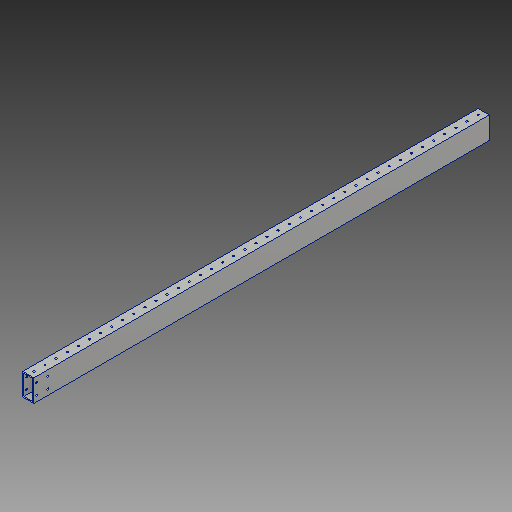
# Autodesk Inventor part: elevator_12''_frame
Saved by Autodesk Inventor 2018 (Build 220112000, 112)
## iProperties
Created: 2018-07-13
Part Number: elevator_12''_frame
Material: Aluminum 6061
Document SubType Name: Modeling
Designer: baoan
Density: 2.7 g/cm^3
Appearance: Aluminum - Flat
Author: baoan
Autodesk Inventor part; units mm, degrees
ref_plane "YZ Plane" through (0, 0, 0) normal (1, 0, 0) x (0, 1, 0)
ref_plane "XZ Plane" through (0, 0, 0) normal (0, 1, 0) x (-1, 0, 0)
ref_plane "XY Plane" through (0, 0, 0) normal (0, 0, 1) x (1, 0, 0)
sketch "Sketch1" plane through (0, 0, 0) normal (0, 0, 1) x (1, 0, 0)
  line L0 (12.7, -25.4) -> (-12.7, -25.4)
  line L1 (-12.7, -25.4) -> (-12.7, 25.4)
  line L2 (-12.7, 25.4) -> (12.7, 25.4)
  line L3 (12.7, 25.4) -> (12.7, -25.4)
  line L4 (12.7, -25.4) -> (-12.7, 25.4) construction
  line L5 (-12.7, -25.4) -> (12.7, 25.4) construction
  line L6 (10.16, -22.86) -> (-10.16, -22.86)
  line L7 (-10.16, -22.86) -> (-10.16, 22.86)
  line L8 (-10.16, 22.86) -> (10.16, 22.86)
  line L9 (10.16, 22.86) -> (10.16, -22.86)
  line L10 (10.16, -22.86) -> (-10.16, 22.86) construction
  line L11 (-10.16, -22.86) -> (10.16, 22.86) construction
  point P0 (0, 0)
  dimension "d0" = 25.4
  dimension "d1" = 50.8
  dimension "d2" = 20.32
  dimension "d3" = 45.72
  constraints: 24 end point, 4 midpoint, 4 parallel, 2 horizontal, 2 perpendicular
  measures "d0" distance of L1.end L2.end
  measures "d1" distance of L0.end L1.end
  measures "d2" distance of L7.end L8.end
  measures "d3" distance of L6.end L7.end
extrude "Extrusion1" add sketch "Sketch1" along normal mid plane 1041.4
sketch "Sketch2" plane through (-12.7, 25.4, 520.7) normal (0, 1, 0) x (1, 0, 0)
  line L0 (0, 0) -> (0, 1041.4) projected
  line L1 (25.4, 0) -> (0, 0) projected
  point P0 (12.7, 520.7)
  point P1 (12.7, 12.7)
  dimension "d6" = 12.7
  dimension "d7" = 12.7
  measures "d6" distance from line of L0 point (12.7, 12.7)
  measures "d7" distance from line of L1 point (12.7, 12.7)
hole "Hole1" at (0, 25.4, 508) direction (0, -1, 0) diameter 4.1402 end through all
pattern_linear "Rectangular Pattern1" count 41 spacing 25.4 along (0, 0, -1) of "Hole1"
sketch "Sketch3" plane through (12.7, -25.4, 520.7) normal (1, 0, 0) x (0, 0, -1)
  line L0 (0, 50.8) -> (1041.4, 50.8) projected
  line L1 (0, 0) -> (0, 50.8) projected
  point P0 (520.7, 25.4)
  point P1 (6.35, 38.1)
  point P2 (6.35, 12.7)
  point P3 (31.75, 38.1)
  point P4 (31.75, 12.7)
  dimension "d18" = 12.7
  dimension "d19" = 25.4
  dimension "d20" = 25.4
  dimension "d22" = 25.4
  dimension "d23" = 6.35
  constraints: 2 vertical alignment, 1 horizontal alignment
  measures "d18" distance from line of L0 point (6.35, 38.1)
  measures "d19" distance of point (6.35, 38.1) point (6.35, 12.7)
  measures "d20" distance of point (31.75, 38.1) point (6.35, 38.1)
  measures "d22" distance of point (31.75, 12.7) point (31.75, 38.1)
  measures "d23" distance from line of L1 point (6.35, 38.1)
hole "Hole2" at (12.7, 12.7, 514.35) at (12.7, -12.7, 514.35) at (12.7, 12.7, 488.95) at (12.7, -12.7, 488.95) direction (-1, 0, 0) diameter 4.1402 end through all
body "Solid1"
